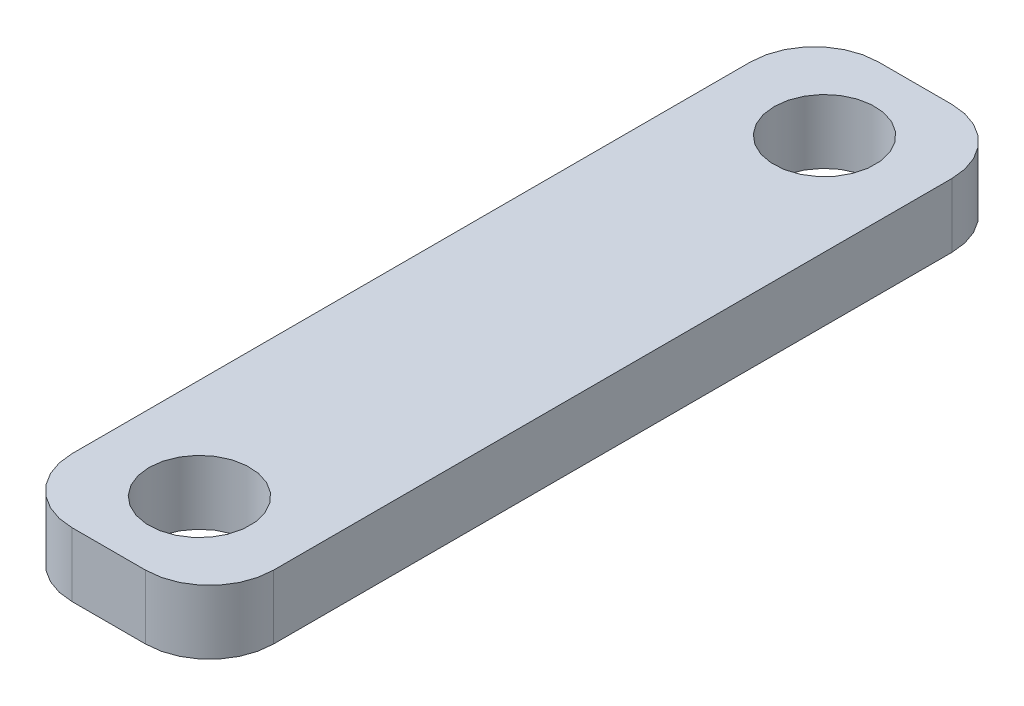
# Autodesk Inventor part: Support_Plate
Saved by Autodesk Inventor 2015 (Build 190159000, 159)
## iProperties
Created: 2014-12-23
Part Number: Support_Plate
Material: Generic
Document SubType Name: Modeling
Designer: Drew
Density: 1 g/cm^3
Appearance: Default
Author: Drew
Autodesk Inventor part; units mm, degrees
ref_plane "YZ Plane" through (0, 0, 0) normal (1, 0, 0) x (0, 1, 0)
ref_plane "XZ Plane" through (0, 0, 0) normal (0, 1, 0) x (-1, 0, 0)
ref_plane "XY Plane" through (0, 0, 0) normal (0, 0, 1) x (1, 0, 0)
sketch "Sketch1" plane through (0, 0, 0) normal (0, 1, 0) x (-1, 0, 0)
  line L0 (-3.65, -40) -> (3.65, -40)
  line L1 (10, -33.65) -> (10, 33.65)
  line L2 (3.65, 40) -> (-3.65, 40)
  line L3 (-10, 33.65) -> (-10, -33.65)
  line L4 (-10, -40) -> (10, 40) construction
  line L5 (10, -40) -> (-10, 40) construction
  line L6 (37.1563, 0) -> (-27.0395, 0)
  circle A0 centre (0, 31) radius 5
  line L7 (0, 56.6322) -> (0, -75.9879)
  circle A1 centre (0, -31) radius 5
  arc A2 (10, 33.65) -> (3.65, 40) centre (3.65, 33.65) ccw
  arc A3 (-3.65, 40) -> (-10, 33.65) centre (-3.65, 33.65) ccw
  arc A4 (-10, -33.65) -> (-3.65, -40) centre (-3.65, -33.65) ccw
  arc A5 (3.65, -40) -> (10, -33.65) centre (3.65, -33.65) ccw
  point P0 (0, 0)
  dimension "d0" = 80
  dimension "d1" = 20
  dimension "d2" = 10
  dimension "d3" = 62
  dimension "d4" = 6.35
  constraints: 16 end point, 9 point on line, 8 point on circle, 8 tangent, 6 centre point, 3 equal radius, 3 horizontal, 2 midpoint, 2 parallel, 2 vertical, 1 perpendicular, 1 symmetric about line, 1 other
  measures "d0" distance of L5.start L4.end
  measures "d1" distance of L4.start L5.start
  measures "d2" diameter of A0
  measures "d3" diameter of A0.centre L6
  measures "d4" radius of A2
extrude "Extrusion1" add sketch "Sketch1" along normal blind 6.35 contours A4 L3 L6 L7 A1 L0 | L7 A1 L6 L1 A5 L0 | L3 A3 L2 L7 A0 L6 | L7 A0 L2 A2 L1 L6
body "Solid1"
